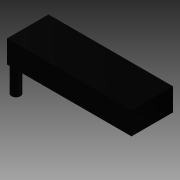
# Autodesk Inventor part: lipol_6000
Saved by Autodesk Inventor 2015 (Build 190159000, 159)
## iProperties
Created: 2015-04-20
Part Number: lipol_6000
Material: Ogólny
Document SubType Name: Modeling
Designer: Marcin
Density: 1 g/cm^3
Appearance: Gładki - czarny
Author: Marcin
Autodesk Inventor part; units mm, degrees
ref_plane "YZ Plane" through (0, 0, 0) normal (1, 0, 0) x (0, 1, 0)
ref_plane "XZ Plane" through (0, 0, 0) normal (0, 1, 0) x (-1, 0, 0)
ref_plane "XY Plane" through (0, 0, 0) normal (0, 0, 1) x (1, 0, 0)
sketch "Szkic1" plane through (0, 0, 0) normal (0, 0, 1) x (1, 0, 0)
  line L0 (-69, -23) -> (69, -23)
  line L1 (69, -23) -> (69, 23)
  line L2 (69, 23) -> (-69, 23)
  line L3 (-69, 23) -> (-69, -23)
  line L4 (-69, -23) -> (69, 23) construction
  line L5 (69, -23) -> (-69, 23) construction
  point P0 (0, 0)
  dimension "d0" = 138
  dimension "d1" = 46
  constraints: 12 end point, 2 midpoint, 2 parallel, 1 horizontal, 1 perpendicular
  measures "d0" distance of L1.end L2.end
  measures "d1" distance of L0.end L1.end
extrude "Wyciągnięcie proste1" add sketch "Szkic1" along normal mid plane 25
sketch "Szkic2" plane through (0, 0, -12.5) normal (0, 0, -1) x (-1, 0, 0)
  line L0 (-69, -23) -> (69, -23) projected
  line L1 (69, -23) -> (69, 23) projected
  line L2 (69, 23) -> (-69, 23) projected
  line L3 (-69, 23) -> (-69, -23) projected
  circle A0 centre (64, -18) radius 5
  circle A1 centre (64, 18) radius 5
  line L4 (-69, -23) -> (69, -23) projected
  line L5 (69, -23) -> (69, 23) projected
  line L6 (69, 23) -> (-69, 23) projected
  point P0 (0, 0)
  dimension "d4" = 10
  dimension "d5" = 10
  constraints: 4 tangent, 2 centre point
  measures "d4" diameter of A0
  measures "d5" diameter of A1
extrude "Wyciągnięcie proste2" add sketch "Szkic2" along normal blind 28 contours A0 | A1
equation "\"d5\" = d4"
